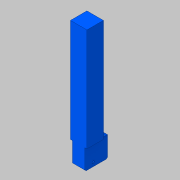
# Autodesk Inventor part: B4-Z
Saved by Autodesk Inventor 2018.1 (Build 221171000, 171)
## iProperties
Created: 2018-06-23
Part Number: B4-Z
Material: Všeobecné
Document SubType Name: Modeling
Designer: PS
Density: 1 g/cm^3
Appearance: Výchozí
Author: PS
Autodesk Inventor part; units mm, degrees
ref_plane "YZ Plane" through (0, 0, 0) normal (1, 0, 0) x (0, 1, 0)
ref_plane "XZ Plane" through (0, 0, 0) normal (0, 1, 0) x (-1, 0, 0)
ref_plane "XY Plane" through (0, 0, 0) normal (0, 0, 1) x (1, 0, 0)
sketch "Náčrt1" plane through (0, 0, 0) normal (0, 0, 1) x (1, 0, 0)
  line L0 (-200, -200) -> (200, -200)
  line L1 (200, -200) -> (200, 200)
  line L2 (200, 200) -> (-200, 200)
  line L3 (-200, 200) -> (-200, -200)
  line L4 (-200, -200) -> (200, 200) construction
  line L5 (200, -200) -> (-200, 200) construction
  point P0 (0, 0)
  dimension "d0" = 400
  dimension "d1" = 400
  constraints: 12 end point, 2 midpoint, 2 parallel, 1 horizontal, 1 perpendicular
  measures "d0" distance of L2.end L1.end
  measures "d1" distance of L1.end L0.end
extrude "Vysunutí1" add sketch "Náčrt1" along normal blind 2500
sketch "Náčrt2" plane through (0, 0, 0) normal (0, 0, -1) x (-1, 0, 0)
  line L0 (200, -200) -> (-200, -200) projected
  line L1 (150, 350) -> (-150, 350)
  line L2 (-150, 350) -> (-150, -200)
  line L3 (-150, -200) -> (150, -200)
  line L4 (150, -200) -> (150, 350)
  line L5 (150, 350) -> (-150, -200) construction
  line L6 (-150, 350) -> (150, -200) construction
  point P0 (0, 75)
  point P1 (0, 0)
  dimension "d15" = 300
  dimension "d16" = 550
  constraints: 12 end point, 2 midpoint, 2 parallel, 1 collinear, 1 horizontal, 1 perpendicular, 1 vertical alignment
  measures "d15" distance of L1.start L1.end
  measures "d16" distance of L3.end L1.start
extrude "Vysunutí2" add sketch "Náčrt2" along normal blind 500
sketch "Náčrt4" plane through (-150, 200, 0) normal (-1, 0, 0) x (0, 0, 1)
  circle A0 centre (-400, -200) radius 25
  line L0 (0, 0) -> (0, -400) projected
  line L1 (0, -200) -> (-500.4879, -200) construction
  line L2 (-500, -400) -> (-500, 150) projected
  dimension "d17" = 50
  dimension "d18" = 100
  constraints: 2 end point, 1 centre point, 1 perpendicular, 1 point on line
  measures "d17" diameter of A0
  measures "d18" distance from line of L2 A0.centre
extrude "Vysunutí4" cut sketch "Náčrt4" against normal blind 500
chamfer "Zkosení2" distance 30 angle 45 2 edges at (0, -200, -500) (0, 350, -500)
